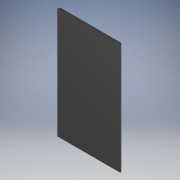
# Autodesk Inventor part: BA03
Saved by Autodesk Inventor 2017 (Build 210142000, 142)
## iProperties
Created: 2018-10-18
Part Number: BA03
Material: ABS Plastic
Document SubType Name: Modeling
Designer: Dell
Density: 1.06 g/cm^3
Appearance: Smooth - Black
Author: Dell
Autodesk Inventor part; units mm, degrees
ref_plane "YZ Plane" through (0, 0, 0) normal (1, 0, 0) x (0, 1, 0)
ref_plane "XZ Plane" through (0, 0, 0) normal (0, 1, 0) x (-1, 0, 0)
ref_plane "XY Plane" through (0, 0, 0) normal (0, 0, 1) x (1, 0, 0)
sketch "Sketch1" plane through (0, 0, 0) normal (0, 0, 1) x (1, 0, 0)
  line L0 (0, 0) -> (292.1, 0)
  line L1 (292.1, 0) -> (292.1, -533.4)
  line L2 (292.1, -533.4) -> (0, -533.4)
  line L3 (0, -533.4) -> (0, 0)
  dimension "d0" = 292.1
  dimension "d1" = 533.4
  constraints: 8 end point, 2 parallel, 1 horizontal, 1 perpendicular
  measures "d0" distance of L1.end L2.end
  measures "d1" distance of L0.end L1.end
extrude "Extrusion1" add sketch "Sketch1" along normal blind 10
sketch "Sketch2" plane through (0, 0, 0) normal (0, 1, 0) x (1, 0, 0)
  line L0 (292.1, -10) -> (0, -10) projected
  line L1 (0, -10) -> (-5.7735, -10)
  line L2 (-5.7735, -10) -> (0, 0)
  line L3 (0, 0) -> (0, -10) projected
  line L4 (0, 0) -> (0, -10) projected
  line L5 (0, -10) -> (0, 0)
  line L6 (292.1, -10) -> (297.8735, -10)
  line L7 (292.1, 0) -> (292.1, -10) projected
  line L8 (297.8735, -10) -> (292.1, 0)
  line L9 (292.1, 0) -> (292.1, -10)
  dimension "d4" = 30
  dimension "d5" = 60
  constraints: 12 end point, 2 collinear, 2 horizontal
  measures "d4" angle of L3 L2
  measures "d5" angle of L6 L8
extrude "Extrusion2" add sketch "Sketch2" against normal blind 533.4
sketch "Sketch3" plane through (0, 0, 10) normal (0, 0, 1) x (1, 0, 0)
  line L0 (0, 0) -> (292.1, 0) construction
  line L1 (292.1, 0) -> (292.1, -533.4) construction
  line L2 (292.1, -533.4) -> (0, -533.4) construction
  line L3 (0, -533.4) -> (0, 0) construction
  circle A0 centre (21.05, -19.05) radius 2.5
  circle A1 centre (21.05, -514.35) radius 2.5
  circle A2 centre (271.05, -514.35) radius 2.5
  circle A3 centre (271.05, -19.05) radius 2.5
  line L4 (21.05, -19.05) -> (271.05, -19.05) construction
  line L5 (271.05, -19.05) -> (271.05, -514.35) construction
  line L6 (271.05, -514.35) -> (21.05, -514.35) construction
  line L7 (21.05, -514.35) -> (21.05, -19.05) construction
  point P0 (146.05, -19.05)
  point P1 (146.05, 0)
  point P2 (271.05, -266.7)
  point P3 (292.1, -266.7)
  dimension "d8" = 5
  dimension "d9" = 5
  dimension "d10" = 5
  dimension "d11" = 5
  dimension "d16" = 21.05
  dimension "d17" = 19.05
  constraints: 8 end point, 4 centre point, 4 midpoint, 2 coincident, 2 parallel, 1 horizontal, 1 horizontal alignment, 1 perpendicular, 1 vertical alignment
  measures "d8" diameter of A0
  measures "d9" diameter of A1
  measures "d10" diameter of A2
  measures "d11" diameter of A3
  measures "d16" distance between parallel lines of L1 L5
  measures "d17" distance between parallel lines of L0 L4
extrude "Extrusion3" cut sketch "Sketch3" against normal through all
body "Solid1"
